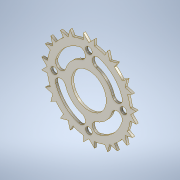
# Autodesk Inventor part: Wood Magnets  (UNI) V1.0.
Saved by Autodesk Inventor 2022.1 (Build 261234020, 234B)
## iProperties
Created: 2022-03-16
Part Number: Wood Magnets  (UNI) V1.0.
Material: Titanium
Document SubType Name: Modeling
Designer: NCai2
Density: 4.51 g/cm^3
Appearance: Titanium
Mass: 5.57938 g
Surface Area: 30.6065 cm^2
Volume: 1.23711 cm^3
Author: NCai2
Autodesk Inventor part; units mm, degrees
ref_plane "YZ Plane" through (0, 0, 0) normal (1, 0, 0) x (0, 1, 0)
ref_plane "XZ Plane" through (0, 0, 0) normal (0, 1, 0) x (-1, 0, 0)
ref_plane "XY Plane" through (0, 0, 0) normal (0, 0, 1) x (1, 0, 0)
sketch "Sketch1" plane through (0, 0, 0) normal (0, 0, 1) x (1, 0, 0)
  circle A0 centre (0, 0) radius 19.05
  circle A1 centre (0, 0) radius 15.875 construction
  circle A2 centre (0, 0) radius 11.1125
  line L0 (0, 0) -> (0, 19.05) construction
  circle A3 centre (0, 15.875) radius 1.5
  line L1 (-1.5875, 10.9985) -> (-1.5875, 18.9837)
  line L2 (1.5875, 10.9985) -> (1.5875, 18.9837)
  circle A4 centre (0, 0) radius 7.9375
  arc A5 (-4.6691, 15.1728) -> (-15.1728, 4.6691) centre (0, 0) ccw
  arc A6 (-15.4746, 3.5428) -> (-11.63, -10.8055) centre (0, 0) ccw
  arc A7 (-10.8055, -11.63) -> (3.5428, -15.4746) centre (0, 0) ccw
  arc A8 (4.6691, -15.1728) -> (15.1728, -4.6691) centre (0, 0) ccw
  arc A9 (15.4746, -3.5428) -> (11.63, 10.8055) centre (0, 0) ccw
  arc A10 (10.8055, 11.63) -> (-3.5428, 15.4746) centre (0, 0) ccw
  line L3 (-1.5875, 18.9837) -> (-1.5875, 21.5237) construction
  line L4 (-1.5875, 21.5237) -> (1.5875, 18.9837) construction
  arc A11 (-15.405, -3.8344) -> (-3.8344, -15.405) centre (0, 0) ccw
  arc A12 (4.6691, -15.1728) -> (15.1728, -4.6691) centre (0, 0) ccw
  arc A13 (15.3341, 4.1088) -> (4.6691, 15.1728) centre (0, 0) ccw
  arc A14 (-4.6691, 15.1728) -> (-15.1728, 4.6691) centre (0, 0) ccw
  line L5 (0, 19.05) -> (-2.54, 19.05) construction
  line L6 (-2.54, 19.05) -> (-2.54, 21.5237) construction
  line L7 (-2.54, 21.5237) -> (0, 21.5237) construction
  line L8 (0, 21.5237) -> (0, 19.05) construction
  line L9 (0, 19.05) -> (-2.54, 21.5237)
  line L10 (-2.54, 18.8799) -> (-2.54, 21.5237)
  line L11 (0, 19.05) -> (2.54, 21.5237)
  line L12 (2.54, 18.8799) -> (2.54, 21.5237)
  line L13 (-9.525, 16.4978) -> (-8.5622, 19.9101)
  line L14 (-7.2402, 17.6205) -> (-8.5622, 19.9101)
  line L15 (-9.525, 16.4978) -> (-12.9616, 17.3701)
  line L16 (-11.6397, 15.0805) -> (-12.9616, 17.3701)
  line L17 (-16.4978, 9.525) -> (-17.3701, 12.9616)
  line L18 (-15.0805, 11.6397) -> (-17.3701, 12.9616)
  line L19 (-16.4978, 9.525) -> (-19.9101, 8.5622)
  line L20 (-17.6205, 7.2402) -> (-19.9101, 8.5622)
  line L21 (-19.05, 0) -> (-21.5237, 2.54)
  line L22 (-18.8799, 2.54) -> (-21.5237, 2.54)
  line L23 (-19.05, 0) -> (-21.5237, -2.54)
  line L24 (-18.8799, -2.54) -> (-21.5237, -2.54)
  line L25 (-16.4978, -9.525) -> (-19.9101, -8.5622)
  line L26 (-17.6205, -7.2402) -> (-19.9101, -8.5622)
  line L27 (-16.4978, -9.525) -> (-17.3701, -12.9616)
  line L28 (-15.0805, -11.6397) -> (-17.3701, -12.9616)
  line L29 (-9.525, -16.4978) -> (-12.9616, -17.3701)
  line L30 (-11.6397, -15.0805) -> (-12.9616, -17.3701)
  line L31 (-9.525, -16.4978) -> (-8.5622, -19.9101)
  line L32 (-7.2402, -17.6205) -> (-8.5622, -19.9101)
  line L33 (0, -19.05) -> (-2.54, -21.5237)
  line L34 (-2.54, -18.8799) -> (-2.54, -21.5237)
  line L35 (0, -19.05) -> (2.54, -21.5237)
  line L36 (2.54, -18.8799) -> (2.54, -21.5237)
  line L37 (9.525, -16.4978) -> (8.5622, -19.9101)
  line L38 (7.2402, -17.6205) -> (8.5622, -19.9101)
  line L39 (9.525, -16.4978) -> (12.9616, -17.3701)
  line L40 (11.6397, -15.0805) -> (12.9616, -17.3701)
  line L41 (16.4978, -9.525) -> (17.3701, -12.9616)
  line L42 (15.0805, -11.6397) -> (17.3701, -12.9616)
  line L43 (16.4978, -9.525) -> (19.9101, -8.5622)
  line L44 (17.6205, -7.2402) -> (19.9101, -8.5622)
  line L45 (19.05, 0) -> (21.5237, -2.54)
  line L46 (18.8799, -2.54) -> (21.5237, -2.54)
  line L47 (19.05, 0) -> (21.5237, 2.54)
  line L48 (18.8799, 2.54) -> (21.5237, 2.54)
  line L49 (16.4978, 9.525) -> (19.9101, 8.5622)
  line L50 (17.6205, 7.2402) -> (19.9101, 8.5622)
  line L51 (16.4978, 9.525) -> (17.3701, 12.9616)
  line L52 (15.0805, 11.6397) -> (17.3701, 12.9616)
  line L53 (9.525, 16.4978) -> (12.9616, 17.3701)
  line L54 (11.6397, 15.0805) -> (12.9616, 17.3701)
  line L55 (9.525, 16.4978) -> (8.5622, 19.9101)
  line L56 (7.2402, 17.6205) -> (8.5622, 19.9101)
  arc A15 (4.6691, 15.1728) -> (3.2684, 10.621) centre (3.9687, 12.8969) ccw
  arc A16 (-3.2684, 10.621) -> (-4.6691, 15.1728) centre (-3.9687, 12.8969) ccw
  arc A17 (-15.1728, 4.6691) -> (-10.621, 3.2684) centre (-12.8969, 3.9688) ccw
  line L57 (-10.9985, 1.5875) -> (-18.9837, 1.5875)
  circle A18 centre (-15.875, 0) radius 1.5
  line L58 (-10.9985, -1.5875) -> (-18.9837, -1.5875)
  arc A19 (-10.621, -3.2684) -> (-15.1728, -4.6691) centre (-12.8969, -3.9688) ccw
  arc A20 (-4.6691, -15.1728) -> (-3.2684, -10.621) centre (-3.9688, -12.8969) ccw
  line L59 (-1.5875, -10.9985) -> (-1.5875, -18.9837)
  circle A21 centre (0, -15.875) radius 1.5
  line L60 (1.5875, -10.9985) -> (1.5875, -18.9837)
  arc A22 (3.2684, -10.621) -> (4.6691, -15.1728) centre (3.9687, -12.8969) ccw
  arc A23 (15.1728, -4.6691) -> (10.621, -3.2684) centre (12.8969, -3.9688) ccw
  line L61 (10.9985, -1.5875) -> (18.9837, -1.5875)
  circle A24 centre (15.875, 0) radius 1.5
  line L62 (10.9985, 1.5875) -> (18.9837, 1.5875)
  arc A25 (10.621, 3.2684) -> (15.1728, 4.6691) centre (12.8969, 3.9688) ccw
  point P0 (1.5875, 14.665)
  point P1 (4.5184, 10.1524)
  point P2 (10.8055, 11.63)
  point P3 (11.63, 10.8055)
  point P4 (-10.8055, -11.63)
  point P5 (-11.63, -10.8055)
  point P6 (-11.6397, 15.0805)
  point P7 (-9.525, 16.4978)
  point P8 (-9.525, 16.4978)
  point P9 (-7.2402, 17.6205)
  point P10 (-17.6205, 7.2402)
  point P11 (-16.4978, 9.525)
  point P12 (-16.4978, 9.525)
  point P13 (-15.0805, 11.6397)
  point P14 (-18.8799, -2.54)
  point P15 (-19.05, 0)
  point P16 (-19.05, 0)
  point P17 (-18.8799, 2.54)
  point P18 (-15.0805, -11.6397)
  point P19 (-16.4978, -9.525)
  point P20 (-16.4978, -9.525)
  point P21 (-17.6205, -7.2402)
  point P22 (-7.2402, -17.6205)
  point P23 (-9.525, -16.4978)
  point P24 (-9.525, -16.4978)
  point P25 (-11.6397, -15.0805)
  point P26 (2.54, -18.8799)
  point P27 (0, -19.05)
  point P28 (0, -19.05)
  point P29 (-2.54, -18.8799)
  point P30 (11.6397, -15.0805)
  point P31 (9.525, -16.4978)
  point P32 (9.525, -16.4978)
  point P33 (7.2402, -17.6205)
  point P34 (17.6205, -7.2402)
  point P35 (16.4978, -9.525)
  point P36 (16.4978, -9.525)
  point P37 (15.0805, -11.6397)
  point P38 (19.05, 0)
  point P39 (19.05, 0)
  point P40 (18.8799, -2.54)
  point P41 (18.8799, 2.54)
  point P42 (15.0805, 11.6397)
  point P43 (16.4978, 9.525)
  point P44 (16.4978, 9.525)
  point P45 (17.6205, 7.2402)
  point P46 (7.2402, 17.6205)
  point P47 (9.525, 16.4978)
  point P48 (9.525, 16.4978)
  point P49 (11.6397, 15.0805)
  point P50 (-14.665, 1.5875)
  point P51 (-1.5875, -14.665)
  point P52 (14.665, -1.5875)
  point P53 (3.2684, -10.621)
  point P54 (10.621, -3.2684)
  point P55 (15.1728, -4.6691)
  point P56 (4.6691, -15.1728)
  point P57 (-3.2684, -10.621)
  point P58 (-4.6691, -15.1728)
  point P59 (-15.1728, -4.6691)
  point P60 (-3.2684, 10.621)
  point P61 (-10.621, 3.2684)
  point P62 (-15.1728, 4.6691)
  point P63 (4.6691, 15.1728)
  point P64 (15.1728, 4.6691)
  point P65 (10.621, 3.2684)
  dimension "d0" = 38.1
  dimension "d1" = 31.75
  dimension "d2" = 22.225
  dimension "d3" = 3
  dimension "d4" = 1.5875
  dimension "d5" = 1.5875
  dimension "d10" = 15.875
  dimension "d13" = 360
  dimension "d15" = 2.54
  dimension "d22" = 2.54
  dimension "d25" = 360
  dimension "d29" = 360
  constraints: 126 end point, 44 point on circle, 25 centre point, 7 point on line, 5 concentric, 5 symmetric about line, 4 coincident, 4 parallel, 4 tangent, 2 perpendicular, 2 vertical, 1 horizontal, 210 other
  measures "d1" diameter of A1
  measures "d2" diameter of A2
  measures "d3" diameter of A3
  measures "d4" distance between parallel lines of L0 L1
  measures "d5" distance between parallel lines of L0 L2
  measures "d10" diameter of A4
  measures "d15" distance of L1.end L3.end
  measures "d22" distance of L6.end L7.end
extrude "Extrusion1" add sketch "Sketch1" along normal blind 1 contours A0 L61 A9 A24 L62 | L45 L46 A0 | A0 L48 L47 | L62 A9 A13 A10 L2 A0 | A0 L60 A22 A8 A23 L61 | L62 A25 A9 | A9 A24 L61 A2 L62 | A0 L49 L50 | L62 A2 A25 | L44 L43 A0 | A23 A2 L61 | A0 L52 L51 | A2 | L41 L42 A0 | A2 L2 A15 | A22 L60 A2 | A0 L53 L54 | A2 L1 A10 A3 L2 | L2 A10 A15 | L40 L39 A0 | L60 A7 A21 L59 A2 | A0 L56 L55 | A2 A16 L1 | A10 A3 L1 A0 L2 | L37 L38 A0 | L60 A0 L59 A7 A21 | L59 A20 A2 | A16 A5 A17 L57 A0 L1 | A0 L11 L12 | A0 L36 L35 | L59 A7 A20 | A2 L57 A17 | A0 L10 L9 | L33 L34 A0 | A19 L58 A2 | A7 L59 A0 L58 A6 A11 | A2 L58 A6 A18 L57 | A19 A6 L58 | A6 A18 L58 A0 L57 | A0 L21 L22 | A0 L13 L14 | L32 L31 A0 | A0 L24 L23 | A0 L16 L15 | L29 L30 A0 | L20 L19 A0 | A0 L25 L26 | L17 L18 A0 | L28 L27 A0
equation "\"OD\" = 38.1"
body "Solid1"
